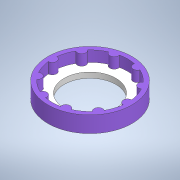
# Autodesk Inventor part: ring
Saved by Autodesk Inventor 2022 (Build 260153000, 153)
## iProperties
Created: 2021-07-18
Part Number: ring
Material: Generic
Document SubType Name: Modeling
Designer: Madhav
Density: 1 g/cm^3
Appearance: Default
Author: Madhav
Autodesk Inventor part; units mm, degrees
ref_plane "YZ Plane" through (0, 0, 0) normal (1, 0, 0) x (0, 1, 0)
ref_plane "XZ Plane" through (0, 0, 0) normal (0, 1, 0) x (-1, 0, 0)
ref_plane "XY Plane" through (0, 0, 0) normal (0, 0, 1) x (1, 0, 0)
sketch "Sketch1" plane through (0, 0, 0) normal (0, 1, 0) x (-1, 0, 0)
  circle A0 centre (0, 0) radius 35
  circle A1 centre (35, 0) radius 4
  circle A2 centre (28.3156, 20.5725) radius 4
  circle A3 centre (10.8156, 33.287) radius 4
  circle A4 centre (-10.8156, 33.287) radius 4
  circle A5 centre (-28.3156, 20.5725) radius 4
  circle A6 centre (-35, 0) radius 4
  circle A7 centre (-28.3156, -20.5725) radius 4
  circle A8 centre (-10.8156, -33.287) radius 4
  circle A9 centre (10.8156, -33.287) radius 4
  circle A10 centre (28.3156, -20.5725) radius 4
  circle A11 centre (0, 0) radius 39
  point P0 (-25.7834, 23.6689)
  point P1 (-14.543, 31.8355)
  point P2 (-6.947, 34.3036)
  point P3 (6.947, 34.3036)
  point P4 (14.543, 31.8355)
  point P5 (25.7834, 23.6689)
  point P6 (30.478, 17.2074)
  point P7 (34.7714, 3.9935)
  point P8 (34.7714, -3.9935)
  point P9 (30.478, -17.2074)
  point P10 (25.7834, -23.6689)
  point P11 (14.543, -31.8355)
  point P12 (6.947, -34.3036)
  point P13 (-6.947, -34.3036)
  point P14 (-14.543, -31.8355)
  point P15 (-25.7834, -23.6689)
  point P16 (-30.478, -17.2074)
  point P17 (-34.7714, -3.9935)
  point P18 (-34.7714, 3.9935)
  point P19 (-30.478, 17.2074)
  dimension "d1" = 70
  dimension "d2" = 8
  dimension "d5" = 360
  dimension "d7" = 78
  constraints: 11 centre point, 2 coincident, 24 other
  measures "d2" diameter of A1
  measures "d7" diameter of A11
extrude "Extrusion1" add sketch "Sketch1" against normal blind 5
extrude "Extrusion2" add sketch "Sketch1" along normal blind 10 contours A0 A1 | A0 A1 | A0 A2 A11 A1 | A1 A11 A10 A0 | A2 A0 | A0 A2 | A10 A0 | A0 A10 | A0 A3 A11 A2 | A11 A9 A0 A10 | A3 A0 | A0 A3 | A3 A0 A4 A11 | A11 A8 A0 A9 | A9 A0 | A0 A9 | A4 A0 | A4 A0 A5 A11 | A11 A7 A0 A8 | A8 A0 | A4 A0 | A5 A0 | A5 A0 A6 A11 | A0 A8 | A11 A6 A0 A7 | A7 A0 | A5 A0 | A6 A0 | A0 A7 | A6 A0
sketch "Sketch2" plane through (0, 0, 0) normal (0, 1, 0) x (1, 0, 0)
  circle A0 centre (0, 0) radius 5
  dimension "d12" = 10
  constraints: 1 centre point, 1 coincident
  measures "d12" diameter of A0
extrude "Extrusion3" cut sketch "Sketch2" against normal blind 10
sketch "Sketch3" plane through (0, -5, 0) normal (0, -1, 0) x (1, 0, 0)
  circle A0 centre (0, 0) radius 24
  dimension "d18" = 48
  constraints: 1 centre point, 1 coincident
  measures "d18" diameter of A0
extrude "Extrusion4" cut sketch "Sketch3" against normal blind 10
body "Solid1"
